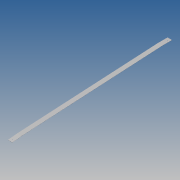
# Autodesk Inventor part: 2p6fs2
Saved by Autodesk Inventor 2014 SP1 (Build 180222100, 222)
## iProperties
Company: HERA Project
Created: 2013-12-11
Part Number: 2p6fs2
Material: Steel
Document SubType Name: Sheet Metal
Designer: David DeBoer
Mass: 1118.84 g
Surface Area: 1199.54 cm^2
Volume: 142.527 cm^3
Density: 7.85 g/cm^3
Description: second furring strip
Appearance: Steel
Sheet Metal Rule: Default
Author: David DeBoer
Autodesk Inventor part; units mm, degrees
ref_plane "YZ Plane" through (0, 0, 0) normal (1, 0, 0) x (0, 1, 0)
ref_plane "XZ Plane" through (0, 0, 0) normal (0, 1, 0) x (-1, 0, 0)
ref_plane "XY Plane" through (0, 0, 0) normal (0, 0, 1) x (1, 0, 0)
sketch "Sketch1" plane through (0, 0, 0) normal (0, 0, 1) x (1, 0, 0)
  line L0 (0, 0) -> (38.1, 0)
  line L1 (38.1, 0) -> (38.1, 1)
  line L2 (38.1, 1) -> (0, 1)
  line L3 (0, 1) -> (0, 0)
  dimension "d0" = 38.1
  dimension "d1" = 1
  constraints: 8 end point, 2 parallel, 1 horizontal, 1 perpendicular
  measures "d0" distance of L0.start L0.end
  measures "d1" distance of L2.end L0.start
extrude "Extrusion1" add sketch "Sketch1" along normal blind 1365
sketch "Sketch2" plane through (0, 1, 0) normal (0, 1, 0) x (1, 0, 0)
  line L0 (38.1, 0) -> (0, 0) projected
  circle A0 centre (19.05, -20) radius 2.2451
  dimension "d4" = 20
  constraints: 1 centre point
  measures "d4" distance from line of A0.centre L0
hole "Hole1" at (19.05, 1, 20) direction (0, -1, 0) diameter 5 end through all
sketch "Sketch3" plane through (0, 1, 0) normal (0, 1, 0) x (1, 0, 0)
  line L0 (38.1, -1365) -> (0, -1365) projected
  circle A0 centre (19.05, -1345) radius 2.2451
  dimension "d12" = 20
  constraints: 1 centre point
  measures "d12" distance from line of L0 A0.centre
hole "Hole2" at (19.05, 1, 1345) direction (0, -1, 0) diameter 5 end through all
sketch "Sketch4" plane through (0, 0, 0) normal (0, -1, 0) x (1, 0, 0)
  circle A0 centre (19.05, 20) radius 2.5 projected
  line L0 (38.1, 0) -> (38.1, 1365) projected
  line L1 (0, 0) -> (0, 1365) projected
  line L2 (0, 80) -> (38.1, 80)
  line L3 (0, 80) -> (1.8993, 80)
  line L4 (0, 80) -> (38.1, 80)
  line L5 (0, 80) -> (38.1, 80) construction
  dimension "d20" = 60
  dimension "d21" = 0
  constraints: 8 end point, 4 point on line, 1 horizontal, 1 perpendicular
  measures "d20" distance from line of L2 A0.centre
  measures "d21" distance between parallel lines of L5 L4
fold "Fold1" angle 3.2 bend radius 1 thickness 1 k factor 0.44 line from (0, 0, 80) to (38.1, 0, 80) line at bend centre moving side (0, 0, 1) folds toward (0, -1, 0)
sketch "Sketch6" plane through (0, -0.0016, 80.0156) normal (0, -0.9984408, -0.0558215) x (1, 0, 0)
  line L0 (38.1, 0) -> (38.1, 1284.9598) projected
  line L1 (0, 0) -> (0, 1284.9598) projected
  circle A0 centre (19.05, 1264.9598) radius 2.5 projected
  line L2 (38.1, 1204.9598) -> (0, 1204.9598)
  line L3 (0, 1204.9598) -> (38.1, 1204.9598)
  line L4 (0, 1204.9598) -> (82.1613, 1204.9598) construction
  point P0 (0, -79.8909)
  dimension "d35" = 60
  dimension "d36" = 0
  constraints: 6 end point, 3 point on line, 1 horizontal, 1 perpendicular
  measures "d35" distance from line of L2 A0.centre
  measures "d36" distance between parallel lines of L3 L4
fold "Fold3" angle 3.2 bend radius 1 thickness 1 k factor 0.44 line from (0, -67.2642, 1283.0966) to (38.1, -67.2642, 1283.0966) line at bend centre moving side (0, -0.0558215, 0.9984408) folds toward (0, -0.9984408, -0.0558215)
sketch "Sketch7" plane through (0, 0.9969, 80.0714) normal (0, 0.9984408, 0.0558215) x (1, 0, 0)
  line L0 (38.1, 0) -> (38.1, -1204.9196) projected
  line L1 (0, 0) -> (0, -1204.9196) projected
  line L2 (0, -602.4598) -> (38.1, -602.4598)
  circle A0 centre (19.05, -452.4598) radius 11.023
  circle A1 centre (19.05, -752.4598) radius 11.023
  point P0 (0, 79.8909)
  dimension "d43" = 150
  constraints: 2 centre point, 2 end point, 2 midpoint, 1 symmetric about line, 1 other
  measures "d43" distance from line of A0.centre L2
hole "Hole3" at (19.05, -41.0066, 831.358) at (19.05, -24.2601, 531.8257) direction (0, -0.9984408, -0.0558215) diameter 1 end through all
equation "\"d1\" = Thickness"
equation "\"d22\" = BendReliefWidth"
equation "\"d23\" = BendReliefDepth"
equation "\"d24\" = MinimumRemnant"
equation "\"d25\" = BendRadius"
equation "\"d26\" = foldAngle"
equation "\"d27\" = BendRadius"
equation "\"d37\" = BendReliefWidth"
equation "\"d38\" = BendReliefDepth"
equation "\"d39\" = MinimumRemnant"
equation "\"d40\" = BendRadius"
equation "\"d41\" = foldAngle"
equation "\"d42\" = BendRadius"
equation "\"d49\" = Thickness"
equation "\"BendRadius\" = Thickness"
equation "\"BendReliefWidth\" = Thickness"
equation "\"BendReliefDepth\" = 0.5 * Thickness"
equation "\"CornerReliefSize\" = 4 * Thickness"
equation "\"MinimumRemnant\" = 2 * Thickness"
equation "\"TransitionRadius\" = BendRadius"
equation "\"JacobiRadiusSize\" = Thickness"
equation "\"GapSize\" = Thickness"
equation "\"foldAngle\" = 3.2deg"
equation "\"Thickness\" = 1"
body "Solid1"
